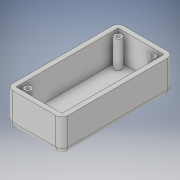
# Autodesk Inventor part: Bottomcase
Saved by Autodesk Inventor 2019 (Build 230136000, 136)
## iProperties
Created: 2019-04-30
Part Number: Bottomcase
Material: Generic
Document SubType Name: Modeling
Designer: Henry
Density: 1 g/cm^3
Appearance: Default
Author: Henry
Autodesk Inventor part; units mm, degrees
ref_plane "YZ Plane" through (0, 0, 0) normal (1, 0, 0) x (0, 1, 0)
ref_plane "XZ Plane" through (0, 0, 0) normal (0, 1, 0) x (-1, 0, 0)
ref_plane "XY Plane" through (0, 0, 0) normal (0, 0, 1) x (1, 0, 0)
sketch "Sketch2" plane through (0, 0, 0) normal (0, 1, 0) x (-1, 0, 0)
  line L0 (0, 0) -> (38.5, 0)
  line L1 (38.5, 0) -> (38.5, -85.5)
  line L2 (38.5, -85.5) -> (0, -85.5)
  line L3 (0, -85.5) -> (0, 0)
  dimension "d5" = 38.5
  dimension "d6" = 85.5
  constraints: 8 end point, 2 parallel, 1 horizontal, 1 perpendicular
  measures "d5" distance of L1.end L2.end
  measures "d6" distance of L0.end L1.end
extrude "Extrusion2" add sketch "Sketch2" along normal blind 4
sketch "Sketch4" plane through (0, 0, 0) normal (0, -1, 0) x (1, 0, 0)
  line L0 (0, 0) -> (4, 0)
  line L1 (4, 0) -> (4, -85.5)
  line L2 (4, -85.5) -> (0, -85.5)
  line L3 (0, -85.5) -> (0, 0)
  line L4 (-38.5, 0) -> (0, 0) projected
  line L5 (-38.5, 0) -> (-42.5, 0)
  line L6 (-42.5, 0) -> (-42.5, -85.5)
  line L7 (-42.5, -85.5) -> (-38.5, -85.5)
  line L8 (-38.5, -85.5) -> (-38.5, 0)
  line L9 (-42.5, -85.5) -> (4, -85.5)
  line L10 (4, -85.5) -> (4, -89.5)
  line L11 (4, -89.5) -> (-42.5, -89.5)
  line L12 (-42.5, -89.5) -> (-42.5, -85.5)
  line L13 (-42.5, 0) -> (4, 0)
  line L14 (4, 0) -> (4, 4)
  line L15 (4, 4) -> (-42.5, 4)
  line L16 (-42.5, 4) -> (-42.5, 0)
  dimension "d13" = 4
  dimension "d14" = 4
  dimension "d15" = 4
  dimension "d16" = 4
  constraints: 32 end point, 8 parallel, 4 horizontal, 4 perpendicular, 2 point on line
  measures "d13" distance of L1.end L2.end
  measures "d14" distance of L7.end L6.end
  measures "d15" distance of L9.end L10.end
  measures "d16" distance of L14.end L13.end
extrude "Extrusion3" add sketch "Sketch4" against normal blind 28 contours L4 L5 L16 L15 L14 L0 | L0 L1 L2 L3 | L2 L10 L11 L12 L7 L9 | L8 L7 L6 L5
fillet "Fillet1" radius 5 4 edges at (-42.5, 0, -42.75) (-19.25, 0, -89.5) (4, 0, -42.75) (-19.25, 0, 4)
fillet "Fillet2" radius 5 2 edges at (-41.0355, 1.4645, 2.5355) (-42.5, 16.5, 4)
fillet "Fillet3" radius 5 6 edges at (2.5355, 1.4645, 2.5355) (4, 16.5, 4) (2.5355, 1.4645, -88.0355) (4, 16.5, -89.5) (-41.0355, 1.4645, -88.0355) (-42.5, 16.5, -89.5)
sketch "Sketch5" plane through (0, 4, 0) normal (0, 1, 0) x (1, 0, 0)
  line L0 (0, 85.5) -> (0, 0) projected
  line L1 (0, 0) -> (-5.0038, 0)
  line L2 (0, 5.0038) -> (0, 0)
  line L3 (0, 85.5) -> (-5.0038, 85.5)
  line L4 (-5.0038, 85.5) -> (-5.0038, 80.4962)
  line L5 (-5.0038, 80.4962) -> (0, 80.4962)
  line L6 (0, 80.4962) -> (0, 85.5)
  circle A0 centre (-5.0038, 80.4962) radius 3
  line L7 (0, 85.5) -> (-38.5, 85.5) projected
  line L8 (-38.5, 85.5) -> (-33.4962, 85.5)
  line L9 (-33.4962, 85.5) -> (-33.4962, 80.4962)
  line L10 (-33.4962, 80.4962) -> (-38.5, 80.4962)
  line L11 (-38.5, 80.4962) -> (-38.5, 85.5)
  circle A1 centre (-33.4962, 80.4962) radius 3
  line L12 (0, 0) -> (-38.5, 0) projected
  line L13 (-38.5, 0) -> (-33.4962, 0)
  line L14 (-33.4962, 0) -> (-33.4962, 5.0038)
  line L15 (-33.4962, 5.0038) -> (-38.5, 5.0038)
  line L16 (-38.5, 5.0038) -> (-38.5, 0)
  circle A2 centre (-33.4962, 5.0038) radius 3
  dimension "d25" = 5.0038
  dimension "d26" = 5.0038
  dimension "d27" = 6
  dimension "d28" = 5.0038
  dimension "d29" = 5.0038
  dimension "d30" = 6
  dimension "d31" = 5.0038
  dimension "d32" = 5.0038
  dimension "d33" = 6
  constraints: 28 end point, 6 parallel, 4 horizontal, 3 centre point, 3 coincident, 3 perpendicular
  measures "d25" distance of L5.end L4.end
  measures "d26" distance of L4.end L3.end
  measures "d27" diameter of A0
  measures "d28" distance of L9.end L10.end
  measures "d29" distance of L8.end L9.end
  measures "d30" diameter of A1
  measures "d31" distance of L15.end L14.end
  measures "d32" distance of L14.end L13.end
  measures "d33" diameter of A2
extrude "Extrusion4" add sketch "Sketch5" along normal blind 23 contours A0 L4 L5 | L5 L4 A0 | A1 L10 L9 | L9 L10 A1 | A2 L15 L14 | L14 L15 A2
sketch "Sketch6" plane through (-33.4962, 27, -5.0038) normal (0, 1, 0) x (1, 0, 0)
  circle A0 centre (0, 0) radius 1.5
  point P0 (33.4962, -5.0038)
  dimension "d36" = 3
  constraints: 1 centre point
  measures "d36" diameter of A0
sketch "Sketch7" plane through (-33.4962, 27, -80.4962) normal (0, 1, 0) x (1, 0, 0)
  circle A0 centre (0, 0) radius 3 projected
  circle A1 centre (0, 0) radius 1.5
  point P0 (33.4962, -80.4962)
  dimension "d37" = 3
  constraints: 1 centre point, 1 coincident
  measures "d37" diameter of A1
sketch "Sketch8" plane through (-5.0038, 27, -80.4962) normal (0, 1, 0) x (1, 0, 0)
  circle A0 centre (0, 0) radius 3 projected
  circle A1 centre (0, 0) radius 1.5
  point P0 (5.0038, -80.4962)
  dimension "d38" = 3
  constraints: 1 centre point, 1 coincident
  measures "d38" diameter of A1
extrude "Extrusion5" cut sketch "Sketch6" against normal blind 15
extrude "Extrusion6" cut sketch "Sketch7" against normal blind 15 contours A1
extrude "Extrusion7" cut sketch "Sketch8" against normal blind 15 contours A1
body "Solid2"
